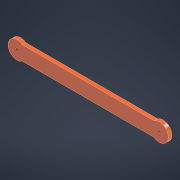
# Autodesk Inventor part: Рычаг_1
Saved by Autodesk Inventor 2021.2 (Build 252289000, 289)
## iProperties
Created: 2021-05-30
Part Number: Рычаг_1
Material: Типовые
Document SubType Name: Modeling
Designer: Admin
Density: 1 g/cm^3
Appearance: Гладкий — светло-оранжевый
Mass: 1443.25 g
Surface Area: 1850.44 cm^2
Volume: 1443.25 cm^3
Author: Admin
Autodesk Inventor part; units mm, degrees
ref_plane "YZ Plane" through (0, 0, 0) normal (1, 0, 0) x (0, 1, 0)
ref_plane "XZ Plane" through (0, 0, 0) normal (0, 1, 0) x (-1, 0, 0)
ref_plane "XY Plane" through (0, 0, 0) normal (0, 0, 1) x (1, 0, 0)
sketch "Эскиз1" plane through (0, 0, 0) normal (0, 0, 1) x (1, 0, 0)
  arc A0 (30, 40) -> (30, -40) centre (0, 0) ccw
  line L0 (30, 40) -> (770, 40)
  line L1 (30, -40) -> (770, -40)
  arc A1 (770, -40) -> (770, 40) centre (800, 0) ccw
  dimension "d0" = 100
  dimension "d1" = 100
  dimension "d3" = 80
  dimension "d4" = 40
  dimension "d5" = 800
  constraints: 4 end point, 4 point on circle, 2 centre point, 2 horizontal, 1 coincident, 1 horizontal alignment
  measures "d0" diameter of A0
  measures "d1" diameter of A1
  measures "d3" distance between parallel lines of L1 L0
  measures "d4" distance from line of point (0, 0) L0
  measures "d5" distance of point (0, 0) A1.centre
extrude "Выдавливание1" add sketch "Эскиз1" along normal blind 20
sketch "Эскиз2" plane through (0, 0, 20) normal (0, 0, 1) x (1, 0, 0)
  arc A0 (770, -40) -> (770, 40) centre (800, 0) ccw projected
  point P0 (0, 0)
  point P1 (0, 0)
  constraints: 2 coincident
hole "Отверстие1" at (0, 0, 20) at (800, 0, 20) direction (0, 0, -1) diameter 18 end through all
